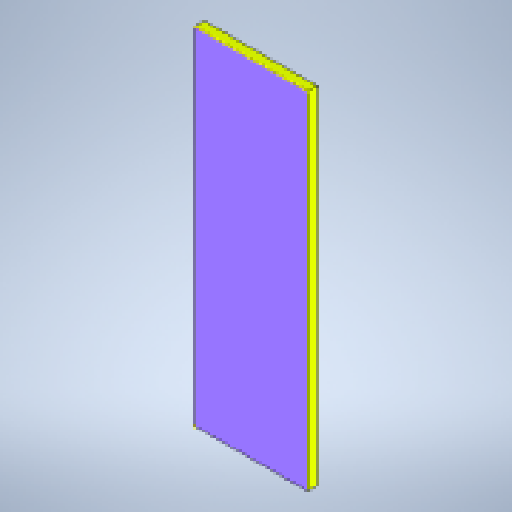
# Autodesk Inventor part: Sandwich Wall 1200 01
Saved by Autodesk Inventor 2025.3 (Build 293356030, 356C)
## iProperties
Created: 2023-05-28
Part Number: Sandwich Wall 1200 01
Material: Generic
Document SubType Name: Modeling
Designer: user
Density: 1 g/cm^3
Appearance: Default
Author: user
Autodesk Inventor part; units mm, degrees
ref_plane "YZ Plane" through (0, 0, 0) normal (1, 0, 0) x (0, 1, 0)
ref_plane "XZ Plane" through (0, 0, 0) normal (0, 1, 0) x (-1, 0, 0)
ref_plane "XY Plane" through (0, 0, 0) normal (0, 0, 1) x (1, 0, 0)
sketch "Sketch1" plane through (0, 0, 0) normal (0, 0, 1) x (1, 0, 0)
  line L0 (0, 0) -> (1200, 0)
  line L1 (1200, 0) -> (1200, 3690)
  line L2 (1200, 3690) -> (0, 3690)
  line L3 (0, 3690) -> (0, 0)
  dimension "d0" = 1200
  dimension "d1" = 3690
  constraints: 8 end point, 2 parallel, 1 horizontal, 1 perpendicular
  measures "d0" distance of L2.end L1.end
  measures "d1" distance of L1.end L0.end
extrude "Extrusion1" add sketch "Sketch1" along normal blind 100
chamfer "Chamfer1" distance 2 angle 45 1 edges at (1200, 1845, 100)
sketch "Sketch3" plane through (0, 0, 100) normal (0, 0, 1) x (1, 0, 0)
  line L0 (1200, 3690) -> (0, 3690) projected
  line L1 (0, 3690) -> (1200, 3434.9321)
  line L2 (1200, 0) -> (1200, 3690) projected
  point P0 (0, 0)
  dimension "d7" = 12
  constraints: 2 end point, 1 point on line
  measures "d7" angle of L1 L0
extrude "Extrusion2" cut sketch "Sketch3" along normal through all both and the other way through all
body "Solid1"
